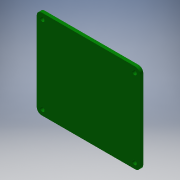
# Autodesk Inventor part: Touchscreen PCB
Saved by Autodesk Inventor 2018 (Build 220112000, 112)
## iProperties
Created: 2018-03-22
Part Number: Touchscreen PCB
Material: Generic
Document SubType Name: Modeling
Designer: brutu
Density: 1 g/cm^3
Appearance: Dark Green
Author: brutu
Autodesk Inventor part; units mm, degrees
ref_plane "YZ Plane" through (0, 0, 0) normal (1, 0, 0) x (0, 1, 0)
ref_plane "XZ Plane" through (0, 0, 0) normal (0, 1, 0) x (-1, 0, 0)
ref_plane "XY Plane" through (0, 0, 0) normal (0, 0, 1) x (1, 0, 0)
sketch "Sketch1" plane through (0, 0, 0) normal (0, 0, 1) x (1, 0, 0)
  line L0 (-29.5, 28) -> (29.5, 28)
  line L1 (32.5, 25) -> (32.5, -25)
  line L2 (29.5, -28) -> (-29.5, -28)
  line L3 (-32.5, -25) -> (-32.5, 25)
  arc A0 (-29.5, 28) -> (-32.5, 25) centre (-29.5, 25) ccw
  arc A1 (32.5, 25) -> (29.5, 28) centre (29.5, 25) ccw
  arc A2 (29.5, -28) -> (32.5, -25) centre (29.5, -25) ccw
  arc A3 (-32.5, -25) -> (-29.5, -28) centre (-29.5, -25) ccw
  point P0 (0, 0)
  point P1 (-32.5, 28)
  point P2 (32.5, 28)
  point P3 (-32.5, -28)
  dimension "d0" = 65
  dimension "d1" = 56
  dimension "d2" = 28
  dimension "d3" = 32.5
  dimension "d4" = 3
  constraints: 8 end point, 8 point on circle, 8 tangent, 6 point on line, 4 centre point, 3 equal radius, 2 parallel, 1 horizontal, 1 perpendicular
  measures "d0" distance of point (-32.5, 28) point (32.5, 28)
  measures "d1" distance of point (-32.5, -28) point (-32.5, 28)
  measures "d2" distance from line of point (0, 0) L0
  measures "d3" distance from line of point (0, 0) L3
  measures "d4" radius of A0
extrude "Extrusion1" add sketch "Sketch1" along normal blind 2
sketch "Sketch2" plane through (0, 0, 0) normal (0, 0, -1) x (-1, 0, 0)
  circle A0 centre (29, 24.5) radius 1.375 projected
  circle A1 centre (-29, 24.5) radius 1.375 projected
  circle A2 centre (-29, -24.5) radius 1.375 projected
  circle A3 centre (29, -24.5) radius 1.375 projected
  point P0 (0, 0)
extrude "Extrusion2" cut sketch "Sketch2" against normal through all
equation "\"d2\" = 0.5 * d1"
equation "\"d3\" = 0.5 * d0"
body "Solid1"
